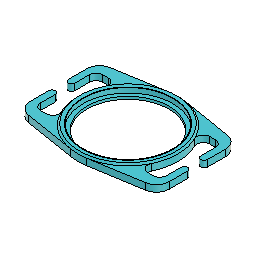
Lens Cap Holder v4 (Autodesk Fusion 360 design; units mm, degrees)
Autodesk Fusion 360 part; units mm, degrees
sketch "Sketch1" plane through (0, 0, 0) normal (1, 0, 0) x (0, 1, 0)
  line L0 (27.5, 0) -> (30.5, 0)
  line L1 (30.5, 0) -> (30.5, 5)
  line L2 (30.5, 5) -> (27.5, 5)
  line L3 (27.5, 5) -> (27.5, 0)
  line L4 (27.5, 4.7) -> (27.2, 4.7)
  line L5 (27.2, 4.7) -> (27.2, 5)
  line L6 (27.2, 5) -> (27.5, 5)
  line L7 (0, 0) -> (0, 12.6279) construction
  dimension "d1" = 27.5
  dimension "d5" = 3
  dimension "d6" = 5
  dimension "d7" = 0.3
  dimension "d8" = 0.3
  constraint horizontal L0
  constraint vertical L1
  constraint horizontal L2
  constraint vertical L3
  constraint coincident L7.start L0
  constraint coincident L3 L4.start
  constraint perpendicular L3 L4
  constraint perpendicular L4 L5
  constraint horizontal L6
  constraint coincident L7.start origin
  constraint vertical L7
  measures "d1" distance of L7.start L3
  measures "d5" distance of L1 L3
  measures "d6" distance of L0 L2
  measures "d7" distance of L4 L6
  measures "d8" distance of L3 L5
revolve "Revolve1" add sketch "Sketch1" angle 360 about axis through (0, 0, 0) along (0, 0, 1)
chamfer "Chamfer1" distance 1 angle 45 1 edges at (-28.436, 11.0293, 5)
sketch "Sketch3" plane through (0, 0, 0) normal (0, 0, 1) x (1, 0, 0)
  line L0 (0, 0) -> (98.0839, 0)
  line L1 (0, 0) -> (73.0788, 0) construction
  circle A0 centre (0, 0) radius 30.5
  line L2 (42.5, 24) -> (42.5, -24)
  line L3 (38.5, 19) -> (38.5, -19)
  line L4 (38.5, 19) -> (23.859, 19)
  line L5 (38.5, -19) -> (23.859, -19)
  circle A1 centre (0, 0) radius 27.5
  line L6 (23.859, 19) -> (-19.8809, 19)
  line L7 (23.859, -19) -> (-23.859, -19)
  line L8 (42.5, 24) -> (4.8873, 30.1059)
  line L9 (42.5, -24) -> (4.8873, -30.1059)
  circle A2 centre (0, 0) radius 33.2
  circle A3 centre (0, 0) radius 27.2
  circle A4 centre (0, 0) radius 25
  dimension "d21" = 42.5
  dimension "d74" = 6
  dimension "d75" = 48
  dimension "d76" = 5
  dimension "d77" = 50
  constraint horizontal L1
  constraint coincident L0.start L1.start
  constraint perpendicular L3 L4
  constraint symmetric L0 L3.start L3.end
  constraint symmetric L0 L4.end L5.end
  constraint coincident A0 L4.end
  constraint horizontal L0
  constraint coincident A1 L6.end
  constraint parallel L4 L6
  constraint coincident A0 L7.end
  constraint parallel L5 L7
  constraint coincident A0 L8.end
  constraint tangent A0 L8
  constraint symmetric L0 L2.start L2.end
  constraint symmetric L0 L8.end L9.end
  constraint concentric A3 A4
  measures "d21" distance of L0.start L2
  measures "d74" distance of A2 A3
  measures "d76" distance of L2.start L4
  measures "d77" diameter of A4
extrude "Extrude2" add sketch "Sketch3" along normal blind 4 contours A0 L4 L8 A2 | A0 L5 L9 A2 | L0 L2 L3 L4 L8 A2 | L0 L2 L3 L5 L9 A2
extrude "Extrude4" add sketch "Sketch3" along normal blind 1.6 contours L0 L6 A3 A4 | L0 L7 A3 A4 | L0 A1 L6 A3 | L0 A1 L7 A3 | L6 A3 A4 | L7 A3 A4 | A1 L6 A3 | A1 L7 A3 | L6 L7 A3 A4 | A1 L6 L7 A3
sketch "Sketch5" plane through (0, 0, 4) normal (0, 0, 1) x (-1, 0, 0)
  line L0 (-52.5, -4) -> (-32.5, -4)
  line L1 (-32.5, -4) -> (-32.5, 4)
  line L2 (-32.5, 4) -> (-52.5, 4)
  line L3 (-52.5, 4) -> (-52.5, -4)
  line L4 (-32.5, 0) -> (0, 0)
  line L5 (-42.5, -24) -> (-4.8873, -30.1059)
  line L6 (-4.8873, 30.1059) -> (-42.5, 24)
  line L7 (-42.5, 24) -> (-42.5, -24)
  arc A0 (-23.859, -19) -> (-4.8873, -30.1059) centre (0, 0) ccw
  line L8 (-23.859, -19) -> (-38.5, -19)
  line L9 (-38.5, -19) -> (-38.5, 19)
  line L10 (-38.5, 19) -> (-23.859, 19)
  arc A1 (-4.8873, 30.1059) -> (-23.859, 19) centre (0, 0) ccw
  dimension "d59" = 8
  dimension "d78" = 32.5
  dimension "d79" = 20
  constraint horizontal L0
  constraint vertical L1
  constraint horizontal L2
  constraint vertical L3
  constraint midpoint L1 L4.start
  constraint coincident L4.end A0.centre
  constraint horizontal L4
  measures "d59" distance of L0.end L1.end
  measures "d78" distance of L1 L4.end
  measures "d79" distance of L0.start L0.end
extrude "Extrude5" cut sketch "Sketch5" against normal blind 8.729 contours L0 L2 L3 L7 | L0 L2 L7 L9 | L0 L1 L2 L9
mirror "Mirror2" about plane through (0, 0, 0) normal (1, 0, 0) of "Extrude2", "Extrude5"
fillet "Fillet6" radius 2 8 edges at (38.5, 4, 2) (42.5, 4, 2) (38.5, -4, 2) (42.5, -4, 2) (-42.5, -4, 2) (-38.5, -4, 2) (-38.5, 4, 2) (-42.5, 4, 2)
fillet "Fillet6" radius 4 8 edges at (-38.5, 19, 2) (-23.859, 19, 2) (-23.859, -19, 2) (-38.5, -19, 2) (23.859, -19, 2) (38.5, -19, 2) (38.5, 19, 2) (23.859, 19, 2)
fillet "Fillet7" radius 8 4 edges at (-42.5, 24, 2) (-42.5, -24, 2) (42.5, 24, 2) (42.5, -24, 2)
equation "d1 = LensDiam / 2"
equation "LensDiam = 55 mm" comment "Lens size"
equation "StrapWidth = 38 mm"
equation "StrapThickness = 2 mm"
equation "d21 = LensDiam / 2 + 15 mm"
equation "d75 = StrapWidth + 10 mm"
equation "d77 = LensDiam - 5 mm"
equation "d78 = LensDiam / 2 + 5 mm"
